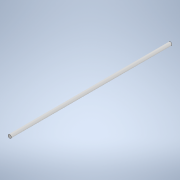
# Autodesk Inventor part: cylinder
Saved by Autodesk Inventor 2020 (Build 240168000, 168)
## iProperties
Created: 2023-03-19
Part Number: cylinder
Material: Generic
Document SubType Name: Modeling
Designer: jcui7
Density: 1 g/cm^3
Appearance: Default
Author: jcui7
Autodesk Inventor part; units mm, degrees
ref_plane "YZ Plane" through (0, 0, 0) normal (1, 0, 0) x (0, 1, 0)
ref_plane "XZ Plane" through (0, 0, 0) normal (0, 1, 0) x (-1, 0, 0)
ref_plane "XY Plane" through (0, 0, 0) normal (0, 0, 1) x (1, 0, 0)
sketch "Sketch1" plane through (0, 0, 0) normal (0, 0, 1) x (1, 0, 0)
  line L0 (0, 0) -> (-22, 0)
  line L1 (-22, 0) -> (-22, -10)
  line L2 (-22, -10) -> (0, -10)
  line L3 (0, -10) -> (0, 0)
  circle A0 centre (-24.1148, -3) radius 1
  line L4 (-22, -6.5922) -> (-24.8297, -3.6992)
  line L5 (-22, -3) -> (-24.1148, -3)
  circle A1 centre (-24.1148, -3) radius 0.5
  line L6 (-22, -0.2647) -> (-24.6952, -2.1857)
  circle A2 centre (-24.1148, -3) radius 0.35
  point P0 (-23.1148, -3)
  point P1 (-23.1148, -3)
  dimension "d0" = 22
  dimension "d1" = 10
  dimension "d2" = 2
  dimension "d3" = 1
  dimension "d4" = 0.7
  constraints: 14 end point, 3 centre point, 2 coincident, 2 horizontal, 2 parallel, 2 point on circle, 2 tangent, 1 perpendicular
  measures "d0" distance of L2.end L1.end
  measures "d1" distance of L1.end L0.end
  measures "d2" diameter of A0
  measures "d3" diameter of A1
  measures "d4" diameter of A2
extrude "Extrusion1" add sketch "Sketch1" against normal blind 34 contours A2
body "Solid1"
